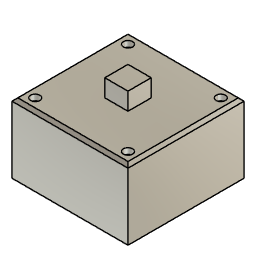
MSE 480 Lab 3 Milling v4 (Autodesk Fusion 360 design; units mm, degrees)
Autodesk Fusion 360 part; units mm, degrees
sketch "Sketch1" plane through (0, 0, 0) normal (0, 0, 1) x (1, 0, 0)
  line L0 (-25.4, 25.4) -> (25.4, 25.4)
  line L1 (25.4, 25.4) -> (25.4, -25.4)
  line L2 (25.4, -25.4) -> (-25.4, -25.4)
  line L3 (-25.4, -25.4) -> (-25.4, 25.4)
  line L4 (-25.4, 25.4) -> (25.4, -25.4) construction
  line L5 (25.4, 25.4) -> (-25.4, -25.4) construction
  dimension "d1" = 50.8
  dimension "d2" = 50.8
  constraint horizontal L0
  constraint perpendicular L0 L1
  constraint parallel L0 L2
  constraint parallel L1 L3
  constraint coincident L4 origin
  constraint coincident L5 origin
  measures "d1" distance of L0.start L2.end
  measures "d2" distance of L0.start L0.end
extrude "Extrude1" add sketch "Sketch1" along normal blind 38.1
sketch "Sketch2" plane through (0, 0, 38.1) normal (0, 0, 1) x (-1, 0, 0)
  line L0 (25.4, 25.4) -> (-25.4, 25.4)
  line L1 (-25.4, 25.4) -> (-25.4, -25.4)
  line L2 (-25.4, -25.4) -> (25.4, -25.4)
  line L3 (25.4, -25.4) -> (25.4, 25.4)
  line L4 (5.08, -5.08) -> (-5.08, -5.08)
  line L5 (-5.08, -5.08) -> (-5.08, 5.08)
  line L6 (-5.08, 5.08) -> (5.08, 5.08)
  line L7 (5.08, 5.08) -> (5.08, -5.08)
  line L8 (5.08, -5.08) -> (-5.08, 5.08) construction
  line L9 (-5.08, -5.08) -> (5.08, 5.08) construction
  line L10 (-25.4, -25.4) -> (25.4, -25.4)
  line L11 (25.4, 25.4) -> (25.4, -25.4)
  line L12 (25.4, 25.4) -> (-25.4, 25.4)
  line L13 (-25.4, -25.4) -> (-25.4, 25.4)
  dimension "d5" = 10.16
  dimension "d6" = 10.16
  constraint horizontal L4
  constraint perpendicular L4 L5
  constraint parallel L4 L6
  constraint parallel L5 L7
  constraint coincident L8 origin
  constraint coincident L9 origin
  constraint coincident L1.end L2.start
  constraint coincident L2.end L3.start
  constraint coincident L0.start L3.end
  constraint coincident L0.end L1.start
  measures "d5" distance of L4.start L6.end
  measures "d6" distance of L4.start L4.end
extrude "Extrude2" cut sketch "Sketch2" against normal blind 7.62
sketch "Sketch3" plane through (0, 0, 30.48) normal (0, 0, 1) x (-1, 0, 0)
  line L0 (-5.08, 5.08) -> (5.08, 5.08)
  line L1 (5.08, 5.08) -> (5.08, -5.08)
  line L2 (5.08, -5.08) -> (-5.08, -5.08)
  line L3 (-5.08, -5.08) -> (-5.08, 5.08)
  line L4 (25.4, 25.4) -> (-25.4, 25.4)
  line L5 (-25.4, 25.4) -> (-25.4, -25.4)
  line L6 (-25.4, -25.4) -> (25.4, -25.4)
  line L7 (25.4, -25.4) -> (25.4, 25.4)
  circle A0 centre (20.32, 20.32) radius 2.032
  circle A1 centre (-20.32, 20.32) radius 2.032
  circle A2 centre (-20.32, -20.32) radius 2.032
  circle A3 centre (20.32, -20.32) radius 2.032
  dimension "d11" = 4.064
  dimension "d13" = 360
  dimension "d14" = 5.08
  dimension "d15" = 5.08
  dimension "d17" = 5.08
  dimension "d18" = 5.08
  dimension "d19" = 5.08
  measures "d11" diameter of A0
  measures "d14" distance of L4 A1.centre
  measures "d15" distance of L4 A0.centre
  measures "d17" distance of L6 A3.centre
  measures "d18" distance of L5 A2.centre
  measures "d19" distance of L7 A0.centre
extrude "Extrude3" cut sketch "Sketch3" against normal blind 2.54 contours A0 | A1 | A2 | A3
sketch "Sketch4" plane through (0, 0, 30.48) normal (0, 0, 1) x (-1, 0, 0)
  circle A0 centre (-20.32, 20.32) radius 2.032
  circle A1 centre (20.32, 20.32) radius 2.032
  circle A2 centre (-20.32, -20.32) radius 2.032
  circle A3 centre (20.32, -20.32) radius 2.032
  line L0 (-5.08, 5.08) -> (5.08, 5.08)
  line L1 (5.08, 5.08) -> (5.08, -5.08)
  line L2 (5.08, -5.08) -> (-5.08, -5.08)
  line L3 (-5.08, -5.08) -> (-5.08, 5.08)
  line L4 (25.4, 25.4) -> (-25.4, 25.4)
  line L5 (-25.4, 25.4) -> (-25.4, -25.4)
  line L6 (-25.4, -25.4) -> (25.4, -25.4)
  line L7 (25.4, -25.4) -> (25.4, 25.4)
  circle A4 centre (20.32, -20.32) radius 1.524
  circle A5 centre (20.32, 20.32) radius 1.524
  circle A6 centre (-20.32, 20.32) radius 1.524
  circle A7 centre (-20.32, -20.32) radius 1.524
  dimension "d22" = 3.048
  dimension "d24" = 360
  constraint concentric A3 A4
  measures "d22" diameter of A4
extrude "Extrude4" cut sketch "Sketch4" against normal blind 20.32 contours A4 | A5 | A6 | A7
chamfer "Chamfer1" distance 1.27 angle 45 4 edges at (0, -25.4, 30.48) (25.4, 0, 30.48) (0, 25.4, 30.48) (-25.4, 0, 30.48)
